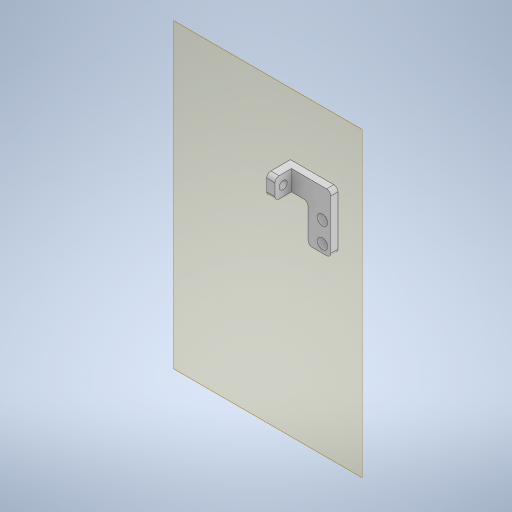
# Autodesk Inventor part: midle-tensioner
Saved by Autodesk Inventor 2024 (Build 280153000, 153)
## iProperties
Created: 2024-04-10
Part Number: midle-tensioner
Material: Generic
Document SubType Name: Modeling
Designer: MaartenGeorgesBuelen
Density: 1 g/cm^3
Appearance: Default
Author: MaartenGeorgesBuelen
## iProperties of the stored document midle-tensioner_3DPrint.ipt
Created: 2024-04-10
Part Number: midle-tensioner_3DPrint
Material: Generic
Document SubType Name: Modeling
Designer: MaartenGeorgesBuelen
Density: 1 g/cm^3
Appearance: Default
Author: MaartenGeorgesBuelen
Autodesk Inventor part; units mm, degrees
ref_plane "YZ Plane" through (0, 0, 0) normal (1, 0, 0) x (0, 1, 0)
ref_plane "XZ Plane" through (0, 0, 0) normal (0, 1, 0) x (-1, 0, 0)
ref_plane "XY Plane" through (0, 0, 0) normal (0, 0, 1) x (1, 0, 0)
ref_plane "Work Plane1" through (0, 0, 0) normal (0, 0, 1) x (1, 0, 0)
sketch "Sketch1" plane through (0, 0, 0) normal (0, 0, 1) x (1, 0, 0)
  circle A0 centre (-18.4345, 53.6439) radius 1.95 projected
  circle A1 centre (-18.4345, 43.6439) radius 1.95 projected
  circle A2 centre (-45.5, -14.5) radius 2.1 projected
  circle A3 centre (-14.5, -14.5) radius 2.1 projected
  circle A4 centre (-14.5, 16.5) radius 2.1 projected
  circle A5 centre (-45.5, 16.5) radius 2.1 projected
  circle A6 centre (-30, 1) radius 13 projected
  arc A7 (30, -41.6762) -> (-30, -41.6762) centre (0, -65) ccw projected
  line L0 (30, -41.6762) -> (30, -22) projected
  line L1 (30, -22) -> (10.1716, -22) projected
  line L2 (10.1716, -22) -> (7, -18.8284) projected
  line L3 (7, -18.8284) -> (7, 20.8284) projected
  line L4 (7, 20.8284) -> (10.1716, 24) projected
  line L5 (10.1716, 24) -> (26, 24) projected
  line L6 (26, 70.5) -> (26, 24) projected
  arc A8 (26, 70.5) -> (5.5, 91) centre (5.5, 70.5) ccw projected
  line L7 (-5.5, 91) -> (5.5, 91) projected
  arc A9 (-5.5, 91) -> (-26, 70.5) centre (-5.5, 70.5) ccw projected
  line L8 (-26, 24) -> (-26, 70.5) projected
  line L9 (-26, 24) -> (-49.8284, 24) projected
  line L10 (-49.8284, 24) -> (-53, 20.8284) projected
  line L11 (-53, 20.8284) -> (-53, -18.8284) projected
  line L12 (-53, -18.8284) -> (-49.8284, -22) projected
  line L13 (-49.8284, -22) -> (-30, -22) projected
  line L14 (-30, -22) -> (-30, -41.6762) projected
  circle A10 centre (18.4345, 43.6439) radius 1.95 projected
  circle A11 centre (18.4345, 53.6439) radius 1.95 projected
  line L15 (11.4345, 57.6439) -> (22.4345, 57.6439)
  line L16 (22.4345, 57.6439) -> (22.4345, 39.6439)
  line L17 (22.4345, 39.6439) -> (11.4345, 39.6439)
  line L18 (11.4345, 39.6439) -> (11.4345, 57.6439)
  circle A12 centre (18.4345, 53.6439) radius 2.45
  circle A13 centre (18.4345, 43.6439) radius 2.45
  line L19 (11.4345, 39.6439) -> (11.4345, 57.6439)
  line L20 (11.4345, 57.6439) -> (22.4345, 57.6439)
  line L21 (22.4345, 57.6439) -> (22.4345, 67.6439)
  line L22 (22.4345, 67.6439) -> (11.4345, 67.6439)
  line L23 (11.4345, 67.6439) -> (11.4345, 57.6439)
  line L24 (9.2719, 63.6439) -> (5.8371, 63.6439)
  line L25 (11.4345, 67.6439) -> (-0.5655, 67.6439)
  line L26 (-0.5655, 67.6439) -> (-0.5655, 57.8782)
  line L27 (-0.5655, 57.8782) -> (11.4345, 57.8782)
  line L28 (11.4345, 57.8782) -> (11.4345, 67.6439)
  point P0 (0, 0)
  point P1 (11.4345, 48.6439)
  dimension "d0" = 4
  dimension "d1" = 4
  dimension "d2" = 4
  dimension "d3" = 7
  dimension "d13" = 0.5
  dimension "d14" = 0.5
  dimension "d27" = 15
  dimension "d28" = 4
  dimension "d29" = 11
  dimension "d30" = 12
  dimension "d31" = 90
  dimension "d32" = 79.8782
  dimension "d33" = 61.6439
  dimension "d34" = 20.7281
  dimension "d35" = 24.1629
  constraints: 28 end point, 6 parallel, 4 horizontal, 3 perpendicular, 2 centre point, 1 midpoint
  measures "d0" distance from line of A11.centre L15
  measures "d1" distance from line of L17 A10.centre
  measures "d2" distance from line of A10.centre L16
  measures "d3" distance from line of A11.centre L18
  measures "d13" radial gap between concentric circles of A11 A12
  measures "d14" radial gap between concentric circles of A10 A13
  measures "d27" distance from line of point (11.435, 48.644) L24
  measures "d28" distance between parallel lines of L22 L24
  measures "d29" distance between parallel lines of L21 L23
  measures "d30" distance of L27.end L26.end
  measures "d31" angle of L1 L19
  measures "d32" distance between parallel lines of L1 L27
  measures "d33" distance from line of L19.start L1
  measures "d34" distance from line of L24.start L0
  measures "d35" distance from line of L24.end L0
extrude "Extrusion1" add sketch "Sketch1" along normal blind 3.5 contours L23 L22 L21 L15 | L15 L16 L17 L18 | L27 L26 L25 L23
sketch "Sketch3" plane through (0, 0, 3.5) normal (0, 0, 1) x (1, 0, 0)
  circle A0 centre (18.4345, 43.6439) radius 2.45 projected
  circle A1 centre (18.4345, 53.6439) radius 2.45 projected
  line L0 (11.4345, 39.6439) -> (22.4345, 39.6439) projected
  line L1 (22.4345, 39.6439) -> (22.4345, 67.6439) projected
  line L2 (22.4345, 67.6439) -> (-0.5655, 67.6439) projected
  line L3 (-0.5655, 67.6439) -> (-0.5655, 57.8782) projected
  line L4 (-0.5655, 57.8782) -> (11.4345, 57.8782) projected
  line L5 (11.4345, 57.8782) -> (11.4345, 39.6439) projected
  line L6 (-0.5655, 67.6439) -> (3.4345, 67.6439)
  line L7 (3.4345, 67.6439) -> (3.4345, 57.8782)
  line L8 (3.4345, 57.8782) -> (-0.5655, 57.8782)
  line L9 (-0.5655, 57.8782) -> (-0.5655, 67.6439)
  point P0 (0, 0)
  dimension "d36" = 4
  constraints: 8 end point, 2 parallel, 1 horizontal, 1 perpendicular, 1 point on line
  measures "d36" distance of L7.end L8.end
extrude "Extrusion3" add sketch "Sketch3" along normal blind 8 contours L4 L3 L2 L7
sketch "Sketch5" plane through (3.4345, 57.8782, 3.5) normal (1, 0, 0) x (0, 0, -1)
  line L0 (0, 9.7657) -> (0, 0) projected
  line L1 (0, 9.7657) -> (-8, 9.7657) projected
  line L2 (-8, 0) -> (-8, 9.7657) projected
  line L3 (0, 0) -> (-8, 0) projected
  line L4 (3.5, -18.2343) -> (3.5, 9.7657) projected
  line L5 (3.5, 9.7657) -> (0, 9.7657) projected
  line L6 (0, -18.2343) -> (0, 9.7657) projected
  line L7 (3.5, -18.2343) -> (0, -18.2343) projected
  circle A0 centre (-4, 4.8829) radius 1.95
  point P0 (3.5, -57.8782)
  dimension "d37" = 3.9
  dimension "d38" = 7.5
  constraints: 1 centre point
  measures "d37" diameter of A0
  measures "d38" distance from line of L4 A0.centre
extrude "Extrusion5" cut sketch "Sketch5" against normal through all contours A0
fillet "Fillet1" radius 2 6 edges at (22.4345, 39.6439, 1.75) (22.4345, 67.6439, 1.75) (11.4345, 57.8782, 1.75) (11.4345, 39.6439, 1.75) (1.4345, 57.8782, 11.5) (1.4345, 67.6439, 11.5)
body "Solid1"
